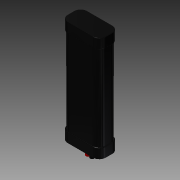
# Autodesk Inventor part: Bateria
Saved by Autodesk Inventor 2015 (Build 190159000, 159)
## iProperties
Created: 2014-06-09
Part Number: Bateria
Material: Genérico
Document SubType Name: Modeling
Designer: Sergio Aguilera
Density: 1 g/cm^3
Appearance: Valor por defecto
Author: Sergio Aguilera
Autodesk Inventor part; units mm, degrees
ref_plane "YZ Plane" through (0, 0, 0) normal (1, 0, 0) x (0, 1, 0)
ref_plane "XZ Plane" through (0, 0, 0) normal (0, 1, 0) x (-1, 0, 0)
ref_plane "XY Plane" through (0, 0, 0) normal (0, 0, 1) x (1, 0, 0)
sketch "Boceto1" plane through (0, 0, 0) normal (0, 1, 0) x (-1, 0, 0)
  line L0 (5.2555, -29.1905) -> (-39.7445, -29.1905)
  line L1 (-39.7445, -29.1905) -> (-39.7445, -134.1905)
  line L2 (-39.7445, -134.1905) -> (5.2555, -134.1905)
  line L3 (5.2555, -134.1905) -> (5.2555, -29.1905)
  point P0 (0, 0)
  dimension "d0" = 45
  dimension "d1" = 105
  constraints: 8 end point, 2 parallel, 1 horizontal, 1 perpendicular
  measures "d0" distance of L2.end L1.end
  measures "d1" distance of L1.end L0.end
extrude "Extrusión1" add sketch "Boceto1" along normal blind 23
sketch "Boceto2" plane through (-5.2555, 0, -29.1905) normal (0, 0, 1) x (1, 0, 0)
  line L0 (-1, 23.5) -> (46, 23.5)
  line L1 (46, 23.5) -> (46, -0.5)
  line L2 (46, -0.5) -> (-1, -0.5)
  line L3 (-1, -0.5) -> (-1, 23.5)
  line L4 (45, 0) -> (45, 23) projected
  line L5 (0, 23) -> (45, 23) projected
  line L6 (0, 0) -> (45, 0) projected
  point P0 (5.2555, 0)
  dimension "d4" = 47
  dimension "d5" = 1
  dimension "d6" = 24
  dimension "d8" = 0.5
  constraints: 8 end point, 2 parallel, 1 horizontal, 1 perpendicular
  measures "d4" distance of L1.end L2.end
  measures "d5" distance between parallel lines of L1 L4
  measures "d6" distance of L0.end L1.end
  measures "d8" distance between parallel lines of L6 L2
extrude "Extrusión2" add sketch "Boceto2" along normal blind 12
sketch "Boceto3" plane through (39.7445, 0, -134.1905) normal (0, 0, -1) x (-1, 0, 0)
  line L0 (-1, 23.5) -> (-1, -0.5) projected
  line L1 (46, 23.5) -> (-1, 23.5) projected
  line L2 (46, -0.5) -> (46, 23.5) projected
  line L3 (-1, -0.5) -> (46, -0.5) projected
  line L4 (-1, 23.5) -> (46, 23.5)
  line L5 (46, 23.5) -> (46, -0.5)
  line L6 (46, -0.5) -> (-1, -0.5)
  line L7 (-1, -0.5) -> (-1, 23.5)
  point P0 (39.7445, 0)
  constraints: 8 end point, 2 parallel, 1 horizontal, 1 perpendicular
extrude "Extrusión3" add sketch "Boceto3" along normal blind 12
sketch "Boceto4" plane through (39.7445, 0, -146.1905) normal (0, 0, -1) x (-1, 0, 0)
  line L0 (-1, 23.5) -> (-1, -0.5) projected
  line L1 (-1, -0.5) -> (46, -0.5) projected
  line L2 (46, 23.5) -> (-1, 23.5) projected
  line L3 (46, -0.5) -> (46, 23.5) projected
  line L4 (4.5, 4.9895) -> (40.5, 4.9895)
  line L5 (40.5, 4.9895) -> (40.5, 18)
  line L6 (40.5, 18) -> (4.5, 18)
  line L7 (4.5, 18) -> (4.5, 4.9895)
  point P0 (39.7445, 0)
  dimension "d13" = 36
  dimension "d14" = 5.5
  dimension "d15" = 5.5
  constraints: 8 end point, 2 parallel, 1 horizontal, 1 perpendicular
  measures "d13" distance of L5.end L6.end
  measures "d14" distance between parallel lines of L3 L5
  measures "d15" distance between parallel lines of L2 L6
extrude "Extrusión4" add sketch "Boceto4" along normal blind 3 contours L7 L6 L5 L4
fillet "Empalme1" radius 8 4 edges at (39.7445, 23, -81.6905) (39.7445, 0, -81.6905) (-5.2555, 23, -81.6905) (-5.2555, 0, -81.6905)
fillet "Empalme2" radius 8 6 edges at (40.7445, 23.5, -23.1905) (40.7445, -0.5, -23.1905) (-6.2555, 23.5, -23.1905) (-6.2555, -0.5, -23.1905) (40.7445, 23.5, -140.1905) (40.7445, -0.5, -140.1905)
fillet "Empalme3" radius 8 2 edges at (-6.2555, 23.5, -140.1905) (-6.2555, -0.5, -140.1905)
fillet "Empalme4" radius 4 4 edges at (35.2445, 4.9895, -147.6905) (35.2445, 18, -147.6905) (-0.7555, 18, -147.6905) (-0.7555, 4.9895, -147.6905)
fillet "Empalme5" radius 0.5 16 edges at (37.4014, 20.6569, -29.1905) (17.2445, 23, -29.1905) (-2.9123, 20.6569, -29.1905) (-5.2555, 11.5, -29.1905) (-2.9123, 2.3431, -29.1905) (17.2445, 0, -29.1905) (37.4014, 2.3431, -29.1905) (39.7445, 11.5, -29.1905) (38.4014, 1.8431, -29.1905) (17.2445, -0.5, -29.1905) (-3.9123, 1.8431, -29.1905) (-6.2555, 11.5, -29.1905) (-3.9123, 21.1569, -29.1905) (17.2445, 23.5, -29.1905) (38.4014, 21.1569, -29.1905) (40.7445, 11.5, -29.1905)
fillet "Empalme6" radius 0.5 40 edges at (34.073, 16.8284, -149.1905) (35.2445, 11.4947, -149.1905) (34.073, 6.161, -149.1905) (17.2445, 4.9895, -149.1905) (0.4161, 6.161, -149.1905) (-0.7555, 11.4947, -149.1905) (0.4161, 16.8284, -149.1905) (17.2445, 18, -149.1905) (0.4161, 16.8284, -146.1905) (-0.7555, 11.4947, -146.1905) (0.4161, 6.161, -146.1905) (17.2445, 4.9895, -146.1905) (34.073, 6.161, -146.1905) (35.2445, 11.4947, -146.1905) (34.073, 16.8284, -146.1905) (17.2445, 18, -146.1905) (17.2445, 23.5, -146.1905) (-3.9123, 21.1569, -146.1905) (-6.2555, 11.5, -146.1905) (-3.9123, 1.8431, -146.1905) (17.2445, -0.5, -146.1905) (38.4014, 1.8431, -146.1905) (40.7445, 11.5, -146.1905) (38.4014, 21.1569, -146.1905) (40.7445, 11.5, -134.1905) (38.4014, 1.8431, -134.1905) (17.2445, -0.5, -134.1905) (-3.9123, 1.8431, -134.1905) (-6.2555, 11.5, -134.1905) (-3.9123, 21.1569, -134.1905) (17.2445, 23.5, -134.1905) (38.4014, 21.1569, -134.1905) (37.4014, 20.6569, -134.1905) (17.2445, 23, -134.1905) (-2.9123, 20.6569, -134.1905) (-5.2555, 11.5, -134.1905) (-2.9123, 2.3431, -134.1905) (17.2445, 0, -134.1905) (37.4014, 2.3431, -134.1905) (39.7445, 11.5, -134.1905)
fillet "Empalme7" radius 0.5 8 edges at (40.7445, 11.5, -17.1905) (38.4014, 1.8431, -17.1905) (17.2445, -0.5, -17.1905) (-3.9123, 1.8431, -17.1905) (-6.2555, 11.5, -17.1905) (-3.9123, 21.1569, -17.1905) (17.2445, 23.5, -17.1905) (38.4014, 21.1569, -17.1905)
sketch "Boceto5" plane through (39.7445, 0, -149.1905) normal (0, 0, -1) x (-1, 0, 0)
  circle A0 centre (25, 11.5) radius 2.5
  line L0 (8.5, 17.5) -> (36.5, 17.5) projected
  line L1 (40, 14) -> (40, 8.9895) projected
  point P0 (39.7445, 0)
  dimension "d26" = 5
  dimension "d29" = 6
  dimension "d30" = 15
  constraints: 1 centre point
  measures "d26" diameter of A0
  measures "d29" distance from line of L0 A0.centre
  measures "d30" distance from line of L1 A0.centre
extrude "Extrusión5" add sketch "Boceto5" along normal blind 9
sketch "Boceto6" plane through (39.7445, 0, -149.1905) normal (0, 0, -1) x (-1, 0, 0)
  circle A0 centre (25, 11.5) radius 2.5 projected
  circle A1 centre (20, 11.5) radius 2.5
  point P0 (39.7445, 0)
  dimension "d33" = 5
  dimension "d34" = 5
  dimension "d35" = 0
  constraints: 1 centre point
  measures "d33" diameter of A1
  measures "d34" distance of A0.centre A1.centre
  measures "d35" vertical distance of A0.centre A1.centre
extrude "Extrusión6" add sketch "Boceto6" along normal blind 9 contours A1
